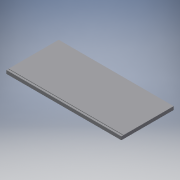
# Autodesk Inventor part: Zijkant 1
Saved by Autodesk Inventor 2018.3 (Build 223284000, 284)
## iProperties
Created: 2020-11-10
Part Number: Zijkant 1
Material: Generic
Document SubType Name: Modeling
Designer: daanv
Density: 1 g/cm^3
Appearance: Default
Author: daanv
Autodesk Inventor part; units mm, degrees
ref_plane "YZ Plane" through (0, 0, 0) normal (1, 0, 0) x (0, 1, 0)
ref_plane "XZ Plane" through (0, 0, 0) normal (0, 1, 0) x (-1, 0, 0)
ref_plane "XY Plane" through (0, 0, 0) normal (0, 0, 1) x (1, 0, 0)
sketch "Sketch1" plane through (0, 0, 0) normal (0, 0, 1) x (1, 0, 0)
  line L0 (0, 0) -> (34.5, 0)
  line L1 (34.5, 0) -> (34.5, 15.7)
  line L2 (34.5, 15.7) -> (0, 15.7)
  line L3 (0, 15.7) -> (0, 0)
  dimension "d0" = 34.5
  dimension "d1" = 15.7
  constraints: 8 end point, 2 parallel, 1 horizontal, 1 perpendicular
  measures "d0" distance of L2.end L1.end
  measures "d1" distance of L1.end L0.end
extrude "Extrusion1" add sketch "Sketch1" along normal blind 1
sketch "Sketch3" plane through (34.5, 0, 0) normal (1, 0, 0) x (0, 0, -1)
  line L0 (-1, 15.7) -> (-1, 0) projected
  line L1 (-1, 0.4) -> (-0.85, 0.4)
  line L2 (-0.85, 0.4) -> (-0.85, 0.7)
  line L3 (-0.85, 0.7) -> (-1, 0.7)
  line L4 (-1, 0.7) -> (-1, 0.4)
  line L5 (0, 0) -> (-1, 0) projected
  dimension "d8" = 0.15
  dimension "d9" = 0.3
  dimension "d12" = 0.4
  constraints: 8 end point, 2 parallel, 1 horizontal, 1 perpendicular, 1 point on line
  measures "d8" distance of L3.end L2.end
  measures "d9" distance of L2.end L1.end
  measures "d12" distance between parallel lines of L1 L5
extrude "Extrusion3" cut sketch "Sketch3" against normal through all
sketch "Sketch4" plane through (0, 0.4, 0.85) normal (0, 0, 1) x (1, 0, 0)
  line L0 (0, 0.3) -> (34.5, 0.3) projected
  line L1 (34.5, 0) -> (34.4, 0)
  line L2 (34.4, 0) -> (34.4, 0.3)
  line L3 (34.4, 0.3) -> (34.5, 0.3)
  line L4 (34.5, 0.3) -> (34.5, 0)
  point P0 (0, -0.4)
  dimension "d13" = 0.1
  constraints: 8 end point, 2 parallel, 1 horizontal, 1 perpendicular, 1 point on line
  measures "d13" distance of L2.end L3.end
extrude "Extrusion4" add sketch "Sketch4" along normal blind 0.15
body "Solid1"
